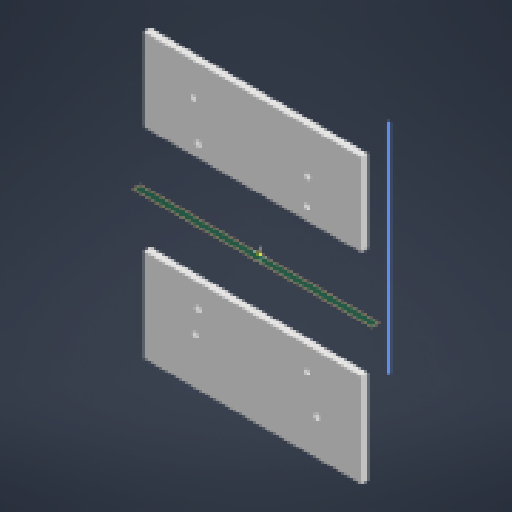
# Autodesk Inventor part: n
Saved by Autodesk Inventor 2026.1 (Build 301233020, 233B)
## iProperties
Created: 2026-01-13
Part Number: n
Material: Generic
Document SubType Name: Modeling
Designer: osama
Density: 1 g/cm^3
Appearance: Default
Author: osama
Autodesk Inventor part; units mm, degrees
ref_plane "YZ Plane" through (0, 0, 0) normal (1, 0, 0) x (0, 1, 0)
ref_plane "XZ Plane" through (0, 0, 0) normal (0, 1, 0) x (-1, 0, 0)
ref_plane "XY Plane" through (0, 0, 0) normal (0, 0, 1) x (1, 0, 0)
sketch "Sketch1" plane through (0, 0, 0) normal (0, 0, 1) x (1, 0, 0)
  line L0 (-48.25, 62.75) -> (48.25, 62.75)
  line L1 (48.25, 62.75) -> (48.25, -62.75)
  line L2 (48.25, -62.75) -> (-48.25, -62.75)
  line L3 (-48.25, -62.75) -> (-48.25, 62.75)
  line L4 (-48.25, 62.75) -> (48.25, -62.75) construction
  line L5 (48.25, 62.75) -> (-48.25, -62.75) construction
  point P0 (0, 0)
  dimension "d0" = 96.5
  dimension "d1" = 125.5
  constraints: 12 end point, 2 midpoint, 2 parallel, 1 horizontal, 1 perpendicular
  measures "d0" distance of L1.end L2.end
  measures "d1" distance of L0.end L1.end
extrude "Extrusion1" add sketch "Sketch1" along normal blind 3
ref_plane "Work Plane2" through (-48.25, 0, 0) normal (0, -1, 0) x (1, 0, 0)
sketch "Sketch3" plane through (0, 0, 0) normal (0, 0, -1) x (-1, 0, 0)
  point P0 (0, 0)
  point P1 (0, 0)
  constraints: 1 coincident
sketch "Sketch4" plane through (0, 0, 0) normal (0, 0, -1) x (-1, 0, 0)
  point P0 (0, 0)
sketch "Sketch5" plane through (0, 0, 0) normal (0, 0, -1) x (-1, 0, 0)
  circle A0 centre (-24.15, 31.81) radius 1.35
  line L0 (-48.25, 62.75) -> (48.25, 62.75) projected
  line L1 (-48.25, -62.75) -> (-48.25, 62.75) projected
  line L2 (-48.25, 62.75) -> (48.25, 62.75) projected
  line L3 (0, 62.75) -> (0, -62.75)
  line L4 (48.25, -62.75) -> (-48.25, -62.75) projected
  circle A1 centre (24.15, 31.81) radius 1.35
  line L5 (-48.25, 0) -> (48.25, 0)
  line L6 (48.25, 62.75) -> (48.25, -62.75) projected
  circle A2 centre (-24.15, -31.81) radius 1.35
  circle A3 centre (24.15, -31.81) radius 1.35
  circle A4 centre (-24.43, 43.61) radius 1.35
  circle A5 centre (26.36, 48.37) radius 1.35
  circle A6 centre (-28.45, -46.87) radius 1.35
  circle A7 centre (25.36, -42.11) radius 1.35
  point P0 (0, 0)
  dimension "d4" = 2.7
  dimension "d6" = 30.94
  dimension "d7" = 24.1
  dimension "d8" = 2.7
  dimension "d9" = 2.7
  dimension "d10" = 2.7
  dimension "d11" = 2.7
  dimension "d12" = 23.82
  dimension "d13" = 19.14
  dimension "d14" = 14.38
  dimension "d15" = 21.89
  dimension "d16" = 19.8
  dimension "d18" = 15.88
  dimension "d19" = 20.64
  dimension "d20" = 22.89
  constraints: 8 centre point, 4 end point, 4 midpoint, 3 symmetric about line, 3 other
  measures "d4" diameter of A0
  measures "d6" distance from line of L0 A0.centre
  measures "d7" distance from line of L1 A0.centre
  measures "d8" diameter of A4
  measures "d9" diameter of A5
  measures "d10" diameter of A6
  measures "d11" diameter of A7
  measures "d12" distance from line of A4.centre L1
  measures "d13" distance from line of L0 A4.centre
  measures "d14" distance from line of L0 A5.centre
  measures "d15" distance from line of L6 A5.centre
  measures "d16" distance from line of L1 A6.centre
  measures "d18" distance from line of L4 A6.centre
  measures "d19" distance from line of L4 A7.centre
  measures "d20" distance from line of L6 A7.centre
extrude "Extrusion2" cut sketch "Sketch5" against normal through all contours A0 | A1 | A2 | A3 | A4 | A5 | A6 | A7
sketch "Sketch6" plane through (0, 0, 0) normal (0, 0, -1) x (-1, 0, 0)
  line L0 (-48.25, -62.75) -> (-48.25, 62.75) projected
  line L1 (48.25, 62.75) -> (48.25, -62.75) projected
  line L2 (-48.25, 26.15) -> (48.25, 26.15)
  line L3 (48.25, 26.15) -> (48.25, -21.475)
  line L4 (48.25, -21.475) -> (-48.25, -21.475)
  line L5 (-48.25, -21.475) -> (-48.25, 26.15)
  line L6 (-48.25, 62.75) -> (48.25, 62.75) projected
  line L7 (48.25, -62.75) -> (-48.25, -62.75) projected
  point P0 (0, 0)
  point P1 (-48.25, -21.475)
  point P2 (48.25, 26.15)
  dimension "d23" = 36.6
  dimension "d24" = 41.275
  constraints: 8 end point, 2 parallel, 2 point on line, 1 horizontal, 1 perpendicular
  measures "d23" distance between parallel lines of L6 L2
  measures "d24" distance between parallel lines of L4 L7
extrude "Extrusion3" cut sketch "Sketch6" against normal blind 10 contours L0 L2 L1 L4
body "Solid1"
